Autodesk Fusion 360 part; units mm, degrees
(part 2 of 3)
  dimension "d347" = 4.5
  dimension "d348" = 4.5
  dimension "d349" = 4.5
  dimension "d350" = 4.5
  dimension "d351" = 4.5
  dimension "d352" = 4.5
  dimension "d353" = 4.5
  dimension "d354" = 4.5
  dimension "d355" = 4.5
  dimension "d356" = 4.5
  dimension "d357" = 4.5
  dimension "d358" = 4.5
  dimension "d359" = 4.5
  dimension "d360" = 4.5
  dimension "d361" = 4.5
  dimension "d362" = 4.5
  dimension "d363" = 4.5
  dimension "d364" = 4.5
  dimension "d365" = 4.5
  dimension "d366" = 4.5
  dimension "d367" = 4.5
  dimension "d368" = 4.5
  dimension "d369" = 4.5
  dimension "d370" = 4.5
  dimension "d371" = 4.5
  dimension "d372" = 4.5
  dimension "d373" = 4.5
  dimension "d374" = 4.5
  dimension "d375" = 4.5
  dimension "d376" = 4.5
  dimension "d377" = 4.5
  dimension "d378" = 4.5
  dimension "d379" = 4.5
  dimension "d380" = 4.5
  dimension "d381" = 4.5
  dimension "d382" = 4.5
  dimension "d383" = 4.5
  dimension "d384" = 4.5
  dimension "d385" = 4.5
  dimension "d386" = 4.5
  dimension "d387" = 4.5
  dimension "d388" = 4.5
  dimension "d389" = 4.5
  dimension "d390" = 4.5
  dimension "d391" = 4.5
  dimension "d392" = 4.5
  dimension "d393" = 4.5
  dimension "d394" = 4.5
  dimension "d395" = 4.5
  dimension "d396" = 4.5
  dimension "d397" = 4.5
  dimension "d398" = 4.5
  dimension "d399" = 4.5
  dimension "d400" = 4.5
  dimension "d401" = 4.5
  dimension "d402" = 4.5
  dimension "d403" = 4.5
  dimension "d404" = 4.5
  dimension "d405" = 4.5
  dimension "d406" = 4.5
  dimension "d407" = 4.5
  dimension "d408" = 4.5
  dimension "d409" = 4.5
  dimension "d410" = 4.5
  dimension "d411" = 4.5
  dimension "d412" = 4.5
  dimension "d413" = 4.5
  dimension "d414" = 4.5
  dimension "d415" = 4.5
  dimension "d416" = 4.5
  dimension "d417" = 4.5
  dimension "d418" = 4.5
  dimension "d419" = 4.5
  dimension "d420" = 4.5
  dimension "d421" = 4.5
  dimension "d422" = 4.5
  dimension "d423" = 4.5
  dimension "d424" = 4.5
  dimension "d425" = 4.5
  dimension "d426" = 4.5
  dimension "d427" = 4.5
  dimension "d428" = 4.5
  dimension "d429" = 4.5
  dimension "d430" = 4.5
  dimension "d431" = 4.5
  dimension "d432" = 4.5
  dimension "d433" = 4.5
  dimension "d434" = 4.5
  dimension "d435" = 4.5
  dimension "d436" = 4.5
  dimension "d437" = 4.5
  dimension "d438" = 4.5
  dimension "d439" = 4.5
  dimension "d440" = 4.5
  dimension "d441" = 4.5
  dimension "d442" = 4.5
  dimension "d443" = 4.5
  dimension "d444" = 4.5
  dimension "d445" = 4.5
  dimension "d446" = 4.5
  dimension "d447" = 4.5
  dimension "d448" = 4.5
  dimension "d449" = 4.5
  dimension "d450" = 4.5
  dimension "d451" = 4.5
  dimension "d452" = 4.5
  dimension "d453" = 4.5
  dimension "d454" = 4.5
  dimension "d455" = 4.5
  dimension "d456" = 4.5
  dimension "d457" = 4.5
  dimension "d458" = 4.5
  dimension "d459" = 4.5
  dimension "d460" = 4.5
  dimension "d461" = 4.5
  dimension "d462" = 4.5
  dimension "d463" = 4.5
  dimension "d464" = 4.5
  dimension "d465" = 4.5
  dimension "d466" = 4.5
  dimension "d467" = 4.5
  dimension "d468" = 4.5
  dimension "d469" = 4.5
  dimension "d470" = 4.5
  dimension "d471" = 4.5
  dimension "d472" = 4.5
  dimension "d473" = 4.5
  dimension "d474" = 4.5
  dimension "d475" = 4.5
  dimension "d476" = 4.5
  dimension "d477" = 4.5
  dimension "d478" = 4.5
  dimension "d479" = 4.5
  dimension "d480" = 4.5
  dimension "d481" = 4.5
  dimension "d482" = 4.5
  dimension "d483" = 4.5
  dimension "d484" = 4.5
  dimension "d485" = 4.5
  dimension "d486" = 4.5
  dimension "d487" = 4.5
  dimension "d488" = 4.5
  dimension "d489" = 4.5
  dimension "d490" = 4.5
  dimension "d491" = 4.5
  dimension "d492" = 4.5
  dimension "d493" = 4.5
  dimension "d494" = 4.5
  dimension "d495" = 4.5
  dimension "d496" = 4.5
  dimension "d497" = 4.5
  dimension "d498" = 4.5
  dimension "d499" = 4.5
  dimension "d500" = 4.5
  dimension "d501" = 4.5
  dimension "d502" = 4.5
  dimension "d503" = 4.5
  dimension "d504" = 4.5
  dimension "d505" = 4.5
  dimension "d506" = 4.5
  dimension "d507" = 4.5
  dimension "d508" = 4.5
  dimension "d509" = 4.5
  dimension "d510" = 4.5
  dimension "d511" = 4.5
  dimension "d512" = 4.5
  dimension "d513" = 4.5
  dimension "d514" = 75
  constraint coincident A0.centre L265.end
  constraint horizontal L0
  constraint vertical L1
  constraint horizontal L2
  constraint vertical L3
  constraint horizontal L6
  constraint vertical L4
  constraint horizontal L7
  constraint vertical L5
  constraint horizontal L12
  constraint vertical L14
  constraint horizontal L9
  constraint vertical L13
  constraint horizontal L15
  constraint vertical L8
  constraint horizontal L11
  constraint vertical L10
  constraint horizontal L20
  constraint vertical L22
  constraint horizontal L17
  constraint vertical L21
  constraint horizontal L23
  constraint vertical L16
  constraint horizontal L19
  constraint vertical L18
  constraint horizontal L28
  constraint vertical L30
  constraint horizontal L25
  constraint vertical L29
  constraint horizontal L31
  constraint vertical L24
  constraint horizontal L27
  constraint vertical L26
  constraint horizontal L36
  constraint vertical L38
  constraint horizontal L33
  constraint vertical L37
  constraint horizontal L39
  constraint vertical L32
  constraint horizontal L35
  constraint vertical L34
  constraint horizontal L44
  constraint vertical L46
  constraint horizontal L41
  constraint vertical L45
  constraint horizontal L47
  constraint vertical L40
  constraint horizontal L43
  constraint vertical L42
  constraint horizontal L52
  constraint vertical L54
  constraint horizontal L49
  constraint vertical L53
  constraint horizontal L55
  constraint vertical L48
  constraint horizontal L51
  constraint vertical L50
  constraint horizontal L86
  constraint vertical L59
  constraint horizontal L74
  constraint vertical L103
  constraint horizontal L65
  constraint vertical L78
  constraint horizontal L110
  constraint vertical L109
  constraint horizontal L94
  constraint vertical L88
  constraint horizontal L80
  constraint vertical L64
  constraint horizontal L99
  constraint vertical L58
  constraint horizontal L98
  constraint vertical L92
  constraint horizontal L87
  constraint vertical L108
  constraint horizontal L76
  constraint vertical L75
  constraint horizontal L84
  constraint vertical L77
  constraint horizontal L104
  constraint vertical L105
  constraint horizontal L111
  constraint vertical L79
  constraint horizontal L106
  constraint vertical L82
  constraint horizontal L96
  constraint vertical L81
  constraint horizontal L83
  constraint vertical L107
  constraint horizontal L97
  constraint vertical L72
  constraint horizontal L60
  constraint vertical L67
  constraint horizontal L93
  constraint vertical L66
  constraint horizontal L71
  constraint vertical L73
  constraint horizontal L101
  constraint vertical L100
  constraint horizontal L85
  constraint vertical L57
  constraint horizontal L69
  constraint vertical L102
  constraint horizontal L95
  constraint vertical L70
  constraint horizontal L56
  constraint vertical L61
  constraint horizontal L68
  constraint vertical L63
  constraint horizontal L89
  constraint vertical L90
  constraint horizontal L62
  constraint vertical L91
  constraint horizontal L223
  constraint vertical L150
  constraint horizontal L220
  constraint vertical L148
  constraint horizontal L222
  constraint vertical L141
  constraint horizontal L219
  constraint vertical L142
  constraint horizontal L217
  constraint vertical L221
  constraint horizontal L144
  constraint vertical L146
  constraint horizontal L151
  constraint vertical L211
  constraint horizontal L145
  constraint vertical L159
  constraint horizontal L186
  constraint vertical L125
  constraint horizontal L163
  constraint vertical L165
  constraint horizontal L169
  constraint vertical L210
  constraint horizontal L191
  constraint vertical L202
  constraint horizontal L137
  constraint vertical L187
  constraint horizontal L173
  constraint vertical L168
  constraint horizontal L204
  constraint vertical L164
  constraint horizontal L128
  constraint vertical L206
  constraint horizontal L215
  constraint vertical L161
  constraint horizontal L201
  constraint vertical L136
  constraint horizontal L162
  constraint vertical L147
  constraint horizontal L149
  constraint vertical L160
  constraint horizontal L209
  constraint vertical L200
  constraint horizontal L194
  constraint vertical L207
  constraint horizontal L196
  constraint vertical L214
  constraint horizontal L195
  constraint vertical L198
  constraint horizontal L130
  constraint vertical L167
  constraint horizontal L216
  constraint vertical L179
  constraint horizontal L182
  constraint vertical L193
  constraint horizontal L213
  constraint vertical L124
  constraint horizontal L114
  constraint vertical L116
  constraint horizontal L158
  constraint vertical L155
  constraint horizontal L120
  constraint vertical L118
  constraint horizontal L152
  constraint vertical L113
  constraint horizontal L112
  constraint vertical L121
  constraint horizontal L115
  constraint vertical L218
  constraint horizontal L140
  constraint vertical L177
  constraint horizontal L143
  constraint vertical L119
  constraint horizontal L170
  constraint vertical L180
  constraint horizontal L212
  constraint vertical L199
  constraint horizontal L178
  constraint vertical L185
  constraint horizontal L139
  constraint vertical L188
  constraint horizontal L129
  constraint vertical L208
  constraint horizontal L171
  constraint vertical L197
  constraint horizontal L203
  constraint vertical L205
  constraint horizontal L181
  constraint vertical L174
  constraint horizontal L122
  constraint vertical L156
  constraint horizontal L127
  constraint vertical L190
  constraint horizontal L117
  constraint vertical L153
  constraint horizontal L157
  constraint vertical L154
  constraint horizontal L131
  constraint vertical L189
  constraint horizontal L184
  constraint vertical L175
  constraint horizontal L126
  constraint vertical L123
  constraint horizontal L138
  constraint vertical L192
  constraint horizontal L135
  constraint vertical L134
  constraint horizontal L172
  constraint vertical L166
  constraint horizontal L176
  constraint vertical L133
  constraint horizontal L132
  constraint vertical L183
  constraint horizontal L439
  constraint vertical L440
  constraint horizontal L441
  constraint vertical L438
  constraint horizontal L281
  constraint vertical L300
  constraint horizontal L283
  constraint vertical L359
  constraint horizontal L289
  constraint vertical L290
  constraint horizontal L293
  constraint vertical L291
  constraint horizontal L240
  constraint vertical L430
  constraint horizontal L249
  constraint vertical L286
  constraint horizontal L434
  constraint vertical L389
  constraint horizontal L326
  constraint vertical L413
  constraint horizontal L421
  constraint vertical L385
  constraint horizontal L333
  constraint vertical L402
  constraint horizontal L376
  constraint vertical L375
  constraint horizontal L379
  constraint vertical L399
  constraint horizontal L428
  constraint vertical L373
  constraint horizontal L361
  constraint vertical L327
  constraint horizontal L356
  constraint vertical L312
  constraint horizontal L323
  constraint vertical L241
  constraint horizontal L314
  constraint vertical L311
  constraint horizontal L315
  constraint vertical L310
  constraint horizontal L239
  constraint vertical L229
  constraint horizontal L253
  constraint vertical L368
  constraint horizontal L230
  constraint vertical L244
  constraint horizontal L237
  constraint vertical L248
  constraint horizontal L391
  constraint vertical L362
  constraint horizontal L369
  constraint vertical L410
  constraint horizontal L403
  constraint vertical L423
  constraint horizontal L435
  constraint vertical L386
  constraint horizontal L437
  constraint vertical L447
  constraint horizontal L442
  constraint vertical L360
  constraint horizontal L287
  constraint vertical L301
  constraint horizontal L277
  constraint vertical L446
  constraint horizontal L282
  constraint vertical L298
  constraint horizontal L279
  constraint vertical L288
  constraint horizontal L228
  constraint vertical L396
  constraint horizontal L235
  constraint vertical L270
  constraint horizontal L426
  constraint vertical L348
  constraint horizontal L401
  constraint vertical L416
  constraint horizontal L432
  constraint vertical L397
  constraint horizontal L336
  constraint vertical L394
  constraint horizontal L387
  constraint vertical L366
  constraint horizontal L324
  constraint vertical L425
  constraint horizontal L343
  constraint vertical L380
  constraint horizontal L388
  constraint vertical L384
  constraint horizontal L352
  constraint vertical L309
  constraint horizontal L357
  constraint vertical L243
  constraint horizontal L254
  constraint vertical L255
  constraint horizontal L313
  constraint vertical L308
  constraint horizontal L227
  constraint vertical L226
  constraint horizontal L245
  constraint vertical L407
  constraint horizontal L233
  constraint vertical L234
  constraint horizontal L242
  constraint vertical L247
  constraint horizontal L427
  constraint vertical L424
  constraint horizontal L415
  constraint vertical L429
  constraint horizontal L371
  constraint vertical L414
  constraint horizontal L372
  constraint vertical L367
  constraint horizontal L445
  constraint vertical L269
  constraint horizontal L224
  constraint vertical L443
  constraint horizontal L280
  constraint vertical L305
  constraint horizontal L284
  constraint vertical L265
  constraint horizontal L296
  constraint vertical L307
  constraint horizontal L295
  constraint vertical L306
  constraint horizontal L236
  constraint vertical L345
  constraint horizontal L329
  constraint vertical L302
  constraint horizontal L404
  constraint vertical L408
  constraint horizontal L349
  constraint vertical L422
  constraint horizontal L342
  constraint vertical L420
  constraint horizontal L355
  constraint vertical L418
  constraint horizontal L365
  constraint vertical L411
  constraint horizontal L383
  constraint vertical L363
  constraint horizontal L395
  constraint vertical L364
  constraint horizontal L381
  constraint vertical L374
  constraint horizontal L334
  constraint vertical L358
  constraint horizontal L350
  constraint vertical L231
  constraint horizontal L264
  constraint vertical L256
  constraint horizontal L261
  constraint vertical L258
  constraint horizontal L419
  constraint vertical L285
  constraint horizontal L431
  constraint vertical L339
  constraint horizontal L250
  constraint vertical L278
  constraint horizontal L272
  constraint vertical L273
  constraint horizontal L340
  constraint vertical L406
  constraint horizontal L398
  constraint vertical L320
  constraint horizontal L331
  constraint vertical L351
  constraint horizontal L405
  constraint vertical L400
  constraint horizontal L268
  constraint vertical L444
  constraint horizontal L225
  constraint vertical L266
  constraint horizontal L276
  constraint vertical L297
  constraint horizontal L275
  constraint vertical L267
  constraint horizontal L292
  constraint vertical L303
  constraint horizontal L294
  constraint vertical L299
  constraint horizontal L238
  constraint vertical L321
  constraint horizontal L354
  constraint vertical L304
  constraint horizontal L392
  constraint vertical L346
  constraint horizontal L344
  constraint vertical L409
  constraint horizontal L316
  constraint vertical L412
  constraint horizontal L332
  constraint vertical L335
  constraint horizontal L390
  constraint vertical L377
  constraint horizontal L370
  constraint vertical L378
  constraint horizontal L433
  constraint vertical L382
  constraint horizontal L417
  constraint vertical L393
  constraint horizontal L318
  constraint vertical L263
  constraint horizontal L347
  constraint vertical L271
  constraint horizontal L257
  constraint vertical L259
  constraint horizontal L260
  constraint vertical L262
  constraint horizontal L325
  constraint vertical L246
  constraint horizontal L436
  constraint vertical L330
  constraint horizontal L232
  constraint vertical L251
  constraint horizontal L252
  constraint vertical L274
  constraint horizontal L322
  constraint vertical L319
  constraint horizontal L328
  constraint vertical L317
  constraint horizontal L338
  constraint vertical L337
  constraint horizontal L341
  constraint vertical L353
  constraint horizontal L663
  constraint vertical L664
  constraint horizontal L665
  constraint vertical L662
  constraint horizontal L505
  constraint vertical L524
  constraint horizontal L507
  constraint vertical L583
  constraint horizontal L513
  constraint vertical L514
  constraint horizontal L517
  constraint vertical L515
  constraint horizontal L464
  constraint vertical L654
  constraint horizontal L473
  constraint vertical L510
  constraint horizontal L658
  constraint vertical L613
  constraint horizontal L550
  constraint vertical L637
  constraint horizontal L645
  constraint vertical L609
  constraint horizontal L557
  constraint vertical L626
  constraint horizontal L600
  constraint vertical L599
  constraint horizontal L603
  constraint vertical L623
  constraint horizontal L652
  constraint vertical L597
  constraint horizontal L585
  constraint vertical L551
  constraint horizontal L580
  constraint vertical L536
  constraint horizontal L547
  constraint vertical L465
  constraint horizontal L538
  constraint vertical L535
  constraint horizontal L539
  constraint vertical L534
  constraint horizontal L463
  constraint vertical L453
  constraint horizontal L477
  constraint vertical L592
  constraint horizontal L454
  constraint vertical L468
  constraint horizontal L461
  constraint vertical L472
  constraint horizontal L615
  constraint vertical L586
  constraint horizontal L593
  constraint vertical L634
  constraint horizontal L627
  constraint vertical L647
  constraint horizontal L659
  constraint vertical L610
  constraint horizontal L661
  constraint vertical L671
  constraint horizontal L666
  constraint vertical L584
  constraint horizontal L511
  constraint vertical L525
  constraint horizontal L501
  constraint vertical L670
  constraint horizontal L506
  constraint vertical L522
  constraint horizontal L503
  constraint vertical L512
  constraint horizontal L452
  constraint vertical L620
  constraint horizontal L459
  constraint vertical L494
  constraint horizontal L650
  constraint vertical L572
  constraint horizontal L625
  constraint vertical L640
  constraint horizontal L656
  constraint vertical L621
  constraint horizontal L560
  constraint vertical L618
  constraint horizontal L611
  constraint vertical L590
  constraint horizontal L548
  constraint vertical L649
  constraint horizontal L567
  constraint vertical L604
  constraint horizontal L612
  constraint vertical L608
  constraint horizontal L576
  constraint vertical L533
  constraint horizontal L581
  constraint vertical L467
  constraint horizontal L478
  constraint vertical L479
  constraint horizontal L537
  constraint vertical L532
  constraint horizontal L451
  constraint vertical L450
  constraint horizontal L469
  constraint vertical L631
  constraint horizontal L457
  constraint vertical L458
  constraint horizontal L466
  constraint vertical L471
  constraint horizontal L651
  constraint vertical L648
  constraint horizontal L639
  constraint vertical L653
  constraint horizontal L595
  constraint vertical L638
  constraint horizontal L596
  constraint vertical L591
  constraint horizontal L669
  constraint vertical L493
  constraint horizontal L448
  constraint vertical L667
  constraint horizontal L504
  constraint vertical L529
  constraint horizontal L508
  constraint vertical L489
  constraint horizontal L520
  constraint vertical L531
  constraint horizontal L519
  constraint vertical L530
  constraint horizontal L460
  constraint vertical L569
  constraint horizontal L553
  constraint vertical L526
  constraint horizontal L628
  constraint vertical L632
  constraint horizontal L573
  constraint vertical L646
  constraint horizontal L566
  constraint vertical L644
  constraint horizontal L579
  constraint vertical L642
  constraint horizontal L589
  constraint vertical L635
  constraint horizontal L607
  constraint vertical L587
  constraint horizontal L619
  constraint vertical L588
  constraint horizontal L605
  constraint vertical L598
  constraint horizontal L558
  constraint vertical L582
  constraint horizontal L574
  constraint vertical L455
  constraint horizontal L488
  constraint vertical L480
  constraint horizontal L485
  constraint vertical L482
  constraint horizontal L643
  constraint vertical L509
  constraint horizontal L655
  constraint vertical L563
  constraint horizontal L474
  constraint vertical L502
  constraint horizontal L496
  constraint vertical L497
  constraint horizontal L564
  constraint vertical L630
  constraint horizontal L622
  constraint vertical L544
  constraint horizontal L555
  constraint vertical L575
  constraint horizontal L629
  constraint vertical L624
  constraint horizontal L492
  constraint vertical L668
  constraint horizontal L449
  constraint vertical L490
  constraint horizontal L500
  constraint vertical L521
  constraint horizontal L499
  constraint vertical L491
  constraint horizontal L516
  constraint vertical L527
  constraint horizontal L518
  constraint vertical L523
  constraint horizontal L462
  constraint vertical L545
  constraint horizontal L578
  constraint vertical L528
  constraint horizontal L616
  constraint vertical L570
  constraint horizontal L568
  constraint vertical L633
  constraint horizontal L540
  constraint vertical L636
  constraint horizontal L556
  constraint vertical L559
  constraint horizontal L614
  constraint vertical L601
  constraint horizontal L594
  constraint vertical L602
  constraint horizontal L657
  constraint vertical L606
  constraint horizontal L641
  constraint vertical L617
  constraint horizontal L542
  constraint vertical L487
  constraint horizontal L571
  constraint vertical L495
  constraint horizontal L481
  constraint vertical L483
  constraint horizontal L484
  constraint vertical L486
  constraint horizontal L549
  constraint vertical L470
  constraint horizontal L660
  constraint vertical L554
  constraint horizontal L456
  constraint vertical L475
  constraint horizontal L476
  constraint vertical L498
  constraint horizontal L546
  constraint vertical L543
  constraint horizontal L552
  constraint vertical L541
  constraint horizontal L562
  constraint vertical L561
  constraint horizontal L565
  constraint vertical L577
  constraint horizontal L887
  constraint vertical L888
  constraint horizontal L889
  constraint vertical L886
  constraint horizontal L729
  constraint vertical L748
  constraint horizontal L731
  constraint vertical L807
  constraint horizontal L737
  constraint vertical L738
  constraint horizontal L741
  constraint vertical L739
  constraint horizontal L688
  constraint vertical L878
  constraint horizontal L697
  constraint vertical L734
  constraint horizontal L882
  constraint vertical L837
  constraint horizontal L774
  constraint vertical L861
  constraint horizontal L869
  constraint vertical L833
  constraint horizontal L781
  constraint vertical L850
  constraint horizontal L824
  constraint vertical L823
  constraint horizontal L827
  constraint vertical L847
  constraint horizontal L876
  constraint vertical L821
  constraint horizontal L809
  constraint vertical L775
  constraint horizontal L804
  constraint vertical L760
  constraint horizontal L771
  constraint vertical L689
  constraint horizontal L762
  constraint vertical L759
  constraint horizontal L763
  constraint vertical L758
  constraint horizontal L687
  constraint vertical L677
  constraint horizontal L701
  constraint vertical L816
  constraint horizontal L678
  constraint vertical L692
  constraint horizontal L685
  constraint vertical L696
  constraint horizontal L839
  constraint vertical L810
  constraint horizontal L817
  constraint vertical L858
  constraint horizontal L851
  constraint vertical L871
  constraint horizontal L883
  constraint vertical L834
  constraint horizontal L885
  constraint vertical L895
  constraint horizontal L890
  constraint vertical L808
  constraint horizontal L735
  constraint vertical L749
  constraint horizontal L725
  constraint vertical L894
  constraint horizontal L730
  constraint vertical L746
  constraint horizontal L727
  constraint vertical L736
  constraint horizontal L676
  constraint vertical L844
  constraint horizontal L683
  constraint vertical L718
  constraint horizontal L874
  constraint vertical L796
  constraint horizontal L849
  constraint vertical L864
  constraint horizontal L880
  constraint vertical L845
  constraint horizontal L784
  constraint vertical L842
  constraint horizontal L835
  constraint vertical L814
  constraint horizontal L772
  constraint vertical L873
  constraint horizontal L791
  constraint vertical L828
  constraint horizontal L836
  constraint vertical L832
  constraint horizontal L800
  constraint vertical L757
  constraint horizontal L805
  constraint vertical L691
  constraint horizontal L702
  constraint vertical L703
  constraint horizontal L761
  constraint vertical L756
  constraint horizontal L675
  constraint vertical L674
  constraint horizontal L693
  constraint vertical L855
  constraint horizontal L681
  constraint vertical L682
  constraint horizontal L690
  constraint vertical L695
  constraint horizontal L875
  constraint vertical L872
  constraint horizontal L863
  constraint vertical L877
  constraint horizontal L819
  constraint vertical L862
  constraint horizontal L820
  constraint vertical L815
  constraint horizontal L893
  constraint vertical L717
  constraint horizontal L672
  constraint vertical L891
  constraint horizontal L728
  constraint vertical L753
  constraint horizontal L732
  constraint vertical L713
  constraint horizontal L744
  constraint vertical L755
  constraint horizontal L743
  constraint vertical L754
  constraint horizontal L684
  constraint vertical L793
  constraint horizontal L777
  constraint vertical L750
  constraint horizontal L852
  constraint vertical L856
  constraint horizontal L797
  constraint vertical L870
  constraint horizontal L790
  constraint vertical L868
  constraint horizontal L803
  constraint vertical L866
  constraint horizontal L813
  constraint vertical L859
  constraint horizontal L831
  constraint vertical L811
  constraint horizontal L843
  constraint vertical L812
  constraint horizontal L829
  constraint vertical L822
  constraint horizontal L782
  constraint vertical L806
  constraint horizontal L798
  constraint vertical L679
  constraint horizontal L712
  constraint vertical L704
  constraint horizontal L709
  constraint vertical L706
  constraint horizontal L867
  constraint vertical L733
  constraint horizontal L879
  constraint vertical L787
  constraint horizontal L698
  constraint vertical L726
  constraint horizontal L720
  constraint vertical L721
  constraint horizontal L788
  constraint vertical L854
  constraint horizontal L846
  constraint vertical L768
  constraint horizontal L779
  constraint vertical L799
  constraint horizontal L853
  constraint vertical L848
  constraint horizontal L716
  constraint vertical L892
  constraint horizontal L673
  constraint vertical L714
  constraint horizontal L724
  constraint vertical L745
  constraint horizontal L723
  constraint vertical L715
  constraint horizontal L740
  constraint vertical L751
  constraint horizontal L742
  constraint vertical L747
  constraint horizontal L686
  constraint vertical L769
  constraint horizontal L802
  constraint vertical L752
  constraint horizontal L840
  constraint vertical L794
  constraint horizontal L792
  constraint vertical L857
  constraint horizontal L764
  constraint vertical L860
  constraint horizontal L780
  constraint vertical L783
  constraint horizontal L838
  constraint vertical L825
  constraint horizontal L818
  constraint vertical L826
  constraint horizontal L881
  constraint vertical L830
  constraint horizontal L865
  constraint vertical L841
  constraint horizontal L766
  constraint vertical L711
  constraint horizontal L795
  constraint vertical L719
  constraint horizontal L705
  constraint vertical L707
  constraint horizontal L708
  constraint vertical L710
  constraint horizontal L773
  constraint vertical L694
  constraint horizontal L884
  constraint vertical L778
  constraint horizontal L680
  constraint vertical L699
  constraint horizontal L700
  constraint vertical L722
  constraint horizontal L770
  constraint vertical L767
  constraint horizontal L776
  constraint vertical L765
  constraint horizontal L786
  constraint vertical L785
  constraint horizontal L789
  constraint vertical L801
  constraint horizontal L935
  constraint vertical L933
  constraint horizontal L940
  constraint vertical L915
  constraint horizontal L896
  constraint vertical L921
  constraint horizontal L919
  constraint vertical L941
  constraint horizontal L928
  constraint vertical L905
  constraint horizontal L918
  constraint vertical L927
  constraint horizontal L925
  constraint vertical L908
  constraint horizontal L909
  constraint vertical L902
  constraint horizontal L907
  constraint vertical L900
  constraint horizontal L926
  constraint vertical L917
  constraint horizontal L912
  constraint vertical L903
  constraint horizontal L901
  constraint vertical L899
  constraint horizontal L913
  constraint vertical L911
  constraint horizontal L897
  constraint vertical L914
  constraint horizontal L898
  constraint vertical L904
  constraint horizontal L906
  constraint vertical L910
  constraint horizontal L932
  constraint vertical L943
  constraint horizontal L934
  constraint vertical L937
  constraint horizontal L936
  constraint vertical L939
  constraint horizontal L931
  constraint vertical L938
  constraint horizontal L946
  constraint vertical L949
  constraint horizontal L929
  constraint vertical L950
  constraint horizontal L922
  constraint vertical L942
  constraint horizontal L924
  constraint vertical L948
  constraint horizontal L945
  constraint vertical L920
  constraint horizontal L951
  constraint vertical L930
  constraint horizontal L944
  constraint vertical L947
  constraint horizontal L923
  constraint vertical L916
  constraint horizontal L991
  constraint vertical L989
  constraint horizontal L996
  constraint vertical L971
  constraint horizontal L952
  constraint vertical L977
  constraint horizontal L975
  constraint vertical L997
  constraint horizontal L984
  constraint vertical L961
  constraint horizontal L974
  constraint vertical L983
  constraint horizontal L981
  constraint vertical L964
  constraint horizontal L965
  constraint vertical L958
  constraint horizontal L963
  constraint vertical L956
  constraint horizontal L982
  constraint vertical L973
  constraint horizontal L968
  constraint vertical L959
  constraint horizontal L957
  constraint vertical L955
  constraint horizontal L969
  constraint vertical L967
  constraint horizontal L953
  constraint vertical L970
  constraint horizontal L954
  constraint vertical L960
  constraint horizontal L962
  constraint vertical L966
  constraint horizontal L988
  constraint vertical L999
  constraint horizontal L990
  constraint vertical L993
  constraint horizontal L992
  constraint vertical L995
  constraint horizontal L987
  constraint vertical L994
  constraint horizontal L1002
  constraint vertical L1005
  constraint horizontal L985
  constraint vertical L1006
  constraint horizontal L978
  constraint vertical L998
  constraint horizontal L980
  constraint vertical L1004
  constraint horizontal L1001
  constraint vertical L976
  constraint horizontal L1007
  constraint vertical L986
  constraint horizontal L1000
  constraint vertical L1003
  constraint horizontal L979
  constraint vertical L972
  constraint horizontal L1008
  constraint vertical L1009
  constraint horizontal L1010
  constraint vertical L1011
  measures "d10" distance of L0.start L0.end
  measures "d11" distance of L0.start L2.end
  measures "d12" distance of L4.start L5.end
  measures "d13" distance of L5.start L5.end
  measures "d14" distance of L12.end L12.start
  measures "d15" distance of L9.end L12.start
  measures "d16" distance of L10.end L8.start
  measures "d17" distance of L10.start L10.end
  measures "d18" distance of L20.end L20.start
  measures "d19" distance of L17.end L20.start
  measures "d20" distance of L18.end L16.start
  measures "d21" distance of L18.start L18.end
  measures "d22" distance of L28.end L28.start
  measures "d23" distance of L25.end L28.start
  measures "d24" distance of L26.end L24.start
  measures "d25" distance of L26.start L26.end
  measures "d26" distance of L36.end L36.start
  measures "d27" distance of L33.end L36.start
  measures "d28" distance of L34.end L32.start
  measures "d29" distance of L34.start L34.end
  measures "d30" distance of L44.end L44.start
  measures "d31" distance of L41.end L44.start
  measures "d32" distance of L42.end L40.start
  measures "d33" distance of L42.start L42.end
  measures "d34" distance of L52.end L52.start
  measures "d35" distance of L49.end L52.start
  measures "d36" distance of L50.end L48.start
  measures "d37" distance of L50.start L50.end
  measures "d38" distance of L59.start L86.start
  measures "d39" distance of L74.end L86.start
  measures "d40" distance of L65.start L65.end
  measures "d41" distance of L109.start L65.start
  measures "d42" distance of L64.end L88.start
  measures "d43" distance of L64.end L64.start
  measures "d44" distance of L58.start L92.end
  measures "d45" distance of L92.start L92.end
  measures "d46" distance of L87.end L75.end
  measures "d47" distance of L75.start L75.end
  measures "d48" distance of L84.start L77.start
  measures "d49" distance of L104.end L84.start
  measures "d50" distance of L82.end L79.start
  measures "d51" distance of L82.start L82.end
  measures "d52" distance of L96.start L81.start
  measures "d53" distance of L83.end L96.start
  measures "d54" distance of L67.end L72.start
  measures "d55" distance of L67.end L60.end
  measures "d56" distance of L73.end L66.start
  measures "d57" distance of L73.end L71.end
  measures "d58" distance of L100.start L57.end
  measures "d59" distance of L57.start L57.end
  measures "d60" distance of L69.end L69.start
  measures "d61" distance of L69.start L70.start
  measures "d62" distance of L56.end L56.start
  measures "d63" distance of L63.start L56.start
  measures "d64" distance of L89.start L89.end
  measures "d65" distance of L89.start L62.end
  measures "d66" distance of L150.start L148.end
  measures "d67" distance of L148.start L148.end
  measures "d68" distance of L142.end L141.start
  measures "d69" distance of L142.start L142.end
  measures "d70" distance of L146.end L217.end
  measures "d71" distance of L146.end L144.end
  measures "d72" distance of L151.end L151.start
  measures "d73" distance of L145.end L151.start
  measures "d74" distance of L125.start L165.end
  measures "d75" distance of L163.end L165.end
  measures "d76" distance of L169.start L169.end
  measures "d77" distance of L191.end L169.start
  measures "d78" distance of L137.start L137.end
  measures "d79" distance of L168.start L137.start
  measures "d80" distance of L204.start L164.start
  measures "d81" distance of L128.end L204.start
  measures "d82" distance of L136.end L161.start
  measures "d83" distance of L136.end L136.start
  measures "d84" distance of L160.end L147.start
  measures "d85" distance of L160.end L149.end
  measures "d86" distance of L200.start L207.end
  measures "d87" distance of L194.end L207.end
  measures "d88" distance of L196.end L196.start
  measures "d89" distance of L196.start L195.end
  measures "d90" distance of L130.end L130.start
  measures "d91" distance of L179.start L130.start
  measures "d92" distance of L124.end L182.end
  measures "d93" distance of L124.end L124.start
  measures "d94" distance of L114.end L114.start
  measures "d95" distance of L155.start L114.start
  measures "d96" distance of L118.start L113.end
  measures "d97" distance of L113.start L113.end
  measures "d98" distance of L112.end L112.start
  measures "d99" distance of L112.start L115.end
  measures "d100" distance of L140.end L119.end
  measures "d101" distance of L119.start L119.end
  measures "d102" distance of L170.end L170.start
  measures "d103" distance of L199.start L170.start
  measures "d104" distance of L178.start L178.end
  measures "d105" distance of L139.end L178.start
  measures "d106" distance of L129.end L129.start
  measures "d107" distance of L171.end L129.start
  measures "d108" distance of L203.end L174.end
  measures "d109" distance of L174.start L174.end
  measures "d110" distance of L122.start L122.end
  measures "d111" distance of L122.start L127.end
  measures "d112" distance of L117.start L117.end
  measures "d113" distance of L117.start L154.start
  measures "d114" distance of L131.end L131.start
  measures "d115" distance of L175.start L131.start
  measures "d116" distance of L126.start L123.start
  measures "d117" distance of L126.start L138.end
  measures "d118" distance of L135.start L134.start
  measures "d119" distance of L135.start L166.start
  measures "d120" distance of L176.start L133.start
  measures "d121" distance of L176.start L132.end
  measures "d122" distance of L439.end L438.end
  measures "d123" distance of L438.start L438.end
  measures "d124" distance of L281.start L281.end
  measures "d125" distance of L283.end L281.start
  measures "d126" distance of L289.start L289.end
  measures "d127" distance of L289.start L291.start
  measures "d128" distance of L240.end L240.start
  measures "d129" distance of L249.end L240.start
  measures "d130" distance of L389.start L413.end
  measures "d131" distance of L326.end L413.end
  measures "d132" distance of L402.end L385.start
  measures "d133" distance of L333.end L402.end
  measures "d134" distance of L376.start L375.start
  measures "d135" distance of L379.end L376.start
  measures "d136" distance of L327.end L373.start
  measures "d137" distance of L327.start L327.end
  measures "d138" distance of L241.end L312.start
  measures "d139" distance of L241.end L241.start
  measures "d140" distance of L310.end L311.start
  measures "d141" distance of L310.end L310.start
  measures "d142" distance of L229.start L239.start
  measures "d143" distance of L253.end L239.start
  measures "d144" distance of L230.end L230.start
  measures "d145" distance of L230.start L237.end
  measures "d146" distance of L362.start L391.start
  measures "d147" distance of L369.end L391.start
  measures "d148" distance of L386.end L403.end
  measures "d149" distance of L386.end L386.start
  measures "d150" distance of L437.end L360.end
  measures "d151" distance of L360.start L360.end
  measures "d152" distance of L287.end L287.start
  measures "d153" distance of L277.end L287.start
  measures "d154" distance of L282.end L282.start
  measures "d155" distance of L282.start L279.end
  measures "d156" distance of L228.end L228.start
  measures "d157" distance of L235.end L228.start
  measures "d158" distance of L348.start L416.end
  measures "d159" distance of L401.end L416.end
  measures "d160" distance of L394.end L397.start
  measures "d161" distance of L336.end L394.end
  measures "d162" distance of L366.start L387.start
  measures "d163" distance of L324.end L387.start
  measures "d164" distance of L343.end L343.start
  measures "d165" distance of L384.start L343.start
  measures "d166" distance of L243.end L309.start
  measures "d167" distance of L243.end L243.start
  measures "d168" distance of L254.start L254.end
  measures "d169" distance of L254.start L308.start
  measures "d170" distance of L226.start L227.start
  measures "d171" distance of L245.end L227.start
  measures "d172" distance of L233.start L233.end
  measures "d173" distance of L233.start L242.end
  measures "d174" distance of L427.start L424.start
  measures "d175" distance of L427.start L415.end
  measures "d176" distance of L367.end L371.end
  measures "d177" distance of L367.end L367.start
  measures "d178" distance of L443.end L269.start
  measures "d179" distance of L224.end L443.end
  measures "d180" distance of A0.centre L280.end
  measures "d181" distance of A0.centre L265.start
  measures "d182" distance of L296.end L296.start
  measures "d183" distance of L295.end L296.start
  measures "d184" distance of L236.end L236.start
  measures "d185" distance of L302.start L236.start
  measures "d186" distance of L404.start L404.end
  measures "d187" distance of L404.start L349.end
  measures "d188" distance of L342.start L342.end
  measures "d189" distance of L342.start L355.end
  measures "d190" distance of L365.end L363.end
  measures "d191" distance of L363.end L363.start
  measures "d192" distance of L364.start L374.end
  measures "d193" distance of L374.end L374.start
  measures "d194" distance of L231.end L334.end
  measures "d195" distance of L231.start L231.end
  measures "d196" distance of L258.end L256.start
  measures "d197" distance of L258.end L258.start
  measures "d198" distance of L285.start L339.end
  measures "d199" distance of L339.end L339.start
  measures "d200" distance of L250.end L250.start
  measures "d201" distance of L272.end L250.start
  measures "d202" distance of L320.end L340.end
  measures "d203" distance of L320.end L320.start
  measures "d204" distance of L331.start L331.end
  measures "d205" distance of L331.start L400.start
  measures "d206" distance of L268.end L266.end
  measures "d207" distance of L225.end L266.end
  measures "d208" distance of L276.end L267.end
  measures "d209" distance of L267.start L267.end
  measures "d210" distance of L292.start L292.end
  measures "d211" distance of L292.start L294.end
  measures "d212" distance of L238.end L238.start
  measures "d213" distance of L238.start L304.start
  measures "d214" distance of L346.start L392.start
  measures "d215" distance of L344.end L392.start
  measures "d216" distance of L316.start L316.end
  measures "d217" distance of L332.end L316.start
  measures "d218" distance of L378.end L377.start
  measures "d219" distance of L378.end L370.end
  measures "d220" distance of L393.end L382.start
  measures "d221" distance of L393.end L393.start
  measures "d222" distance of L271.end L263.start
  measures "d223" distance of L271.end L271.start
  measures "d224" distance of L257.end L257.start
  measures "d225" distance of L260.end L257.start
  measures "d226" distance of L246.start L325.start
  measures "d227" distance of L330.start L325.start
  measures "d228" distance of L232.end L232.start
  measures "d229" distance of L232.start L252.end
  measures "d230" distance of L319.start L317.end
  measures "d231" distance of L317.start L317.end
  measures "d232" distance of L337.start L338.start
  measures "d233" distance of L341.end L338.start
  measures "d234" distance of L0.end L0.start
  measures "d235" distance of L2.end L0.start
  measures "d236" distance of L5.end L4.start
  measures "d237" distance of L5.start L5.end
  measures "d238" distance of L12.start L12.end
  measures "d239" distance of L12.start L9.end
  measures "d240" distance of L8.start L10.end
  measures "d241" distance of L10.start L10.end
  measures "d242" distance of L20.end L20.start
  measures "d243" distance of L17.end L20.start
  measures "d244" distance of L18.end L16.start
  measures "d245" distance of L18.start L18.end
  measures "d246" distance of L28.start L28.end
  measures "d247" distance of L25.end L28.start
  measures "d248" distance of L26.end L24.start
  measures "d249" distance of L26.start L26.end
  measures "d250" distance of L36.start L36.end
  measures "d251" distance of L36.start L33.end
  measures "d252" distance of L34.end L32.start
  measures "d253" distance of L34.end L34.start
  measures "d254" distance of L44.end L44.start
  measures "d255" distance of L41.end L44.start
  measures "d256" distance of L40.start L42.end
  measures "d257" distance of L42.end L42.start
  measures "d258" distance of L52.end L52.start
  measures "d259" distance of L49.end L52.start
  measures "d260" distance of L50.end L48.start
  measures "d261" distance of L50.end L50.start
  measures "d262" distance of L59.start L86.start
  measures "d263" distance of L74.end L86.start
  measures "d264" distance of L65.end L65.start
  measures "d265" distance of L109.start L65.start
  measures "d266" distance of L88.start L64.end
  measures "d267" distance of L64.end L64.start
  measures "d268" distance of L58.start L92.end
  measures "d269" distance of L92.start L92.end
  measures "d270" distance of L87.end L75.end
  measures "d271" distance of L75.start L75.end
  measures "d272" distance of L84.start L77.start
  measures "d273" distance of L104.end L84.start
  measures "d274" distance of L79.start L82.end
  measures "d275" distance of L82.start L82.end
  measures "d276" distance of L81.start L96.start
  measures "d277" distance of L83.end L96.start
  measures "d278" distance of L67.end L72.start
  measures "d279" distance of L67.end L60.end
  measures "d280" distance of L73.end L66.start
  measures "d281" distance of L73.end L71.end
  measures "d282" distance of L100.start L57.end
  measures "d283" distance of L57.start L57.end
  measures "d284" distance of L69.start L69.end
  measures "d285" distance of L69.start L70.start
  measures "d286" distance of L56.start L56.end
  measures "d287" distance of L56.start L63.start
  measures "d288" distance of L89.start L89.end
  measures "d289" distance of L89.start L62.end
  measures "d290" distance of L148.end L150.start
  measures "d291" distance of L148.start L148.end
  measures "d292" distance of L142.end L141.start
  measures "d293" distance of L142.end L142.start
  measures "d294" distance of L217.end L146.end
  measures "d295" distance of L144.end L146.end
  measures "d296" distance of L151.end L151.start
  measures "d297" distance of L145.end L151.start
  measures "d298" distance of L165.end L125.start
  measures "d299" distance of L165.end L163.end
  measures "d300" distance of L169.start L169.end
  measures "d301" distance of L169.start L191.end
  measures "d302" distance of L137.end L137.start
  measures "d303" distance of L137.start L168.start
  measures "d304" distance of L164.start L204.start
  measures "d305" distance of L204.start L128.end
  measures "d306" distance of L136.end L161.start
  measures "d307" distance of L136.start L136.end
  measures "d308" distance of L160.end L147.start
  measures "d309" distance of L160.end L149.end
  measures "d310" distance of L200.start L207.end
  measures "d311" distance of L207.end L194.end
  measures "d312" distance of L196.end L196.start
  measures "d313" distance of L195.end L196.start
  measures "d314" distance of L130.start L130.end
  measures "d315" distance of L130.start L179.start
  measures "d316" distance of L124.end L182.end
  measures "d317" distance of L124.end L124.start
  measures "d318" distance of L114.end L114.start
  measures "d319" distance of L155.start L114.start
  measures "d320" distance of L118.start L113.end
  measures "d321" distance of L113.start L113.end
  measures "d322" distance of L112.start L112.end
  measures "d323" distance of L112.start L115.end
  measures "d324" distance of L140.end L119.end
  measures "d325" distance of L119.end L119.start
  measures "d326" distance of L170.end L170.start
  measures "d327" distance of L199.start L170.start
  measures "d328" distance of L178.start L178.end
  measures "d329" distance of L139.end L178.start
  measures "d330" distance of L129.start L129.end
  measures "d331" distance of L129.start L171.end
  measures "d332" distance of L174.end L203.end
  measures "d333" distance of L174.end L174.start
  measures "d334" distance of L122.start L122.end
  measures "d335" distance of L122.start L127.end
  measures "d336" distance of L117.end L117.start
  measures "d337" distance of L154.start L117.start
  measures "d338" distance of L131.end L131.start
  measures "d339" distance of L175.start L131.start
  measures "d340" distance of L123.start L126.start
  measures "d341" distance of L126.start L138.end
  measures "d342" distance of L134.start L135.start
  measures "d343" distance of L166.start L135.start
  measures "d344" distance of L133.start L176.start
  measures "d345" distance of L132.end L176.start
  measures "d346" distance of L887.end L886.end
  measures "d347" distance of L886.start L886.end
  measures "d348" distance of L729.start L729.end
  measures "d349" distance of L731.end L729.start
  measures "d350" distance of L737.start L737.end
  measures "d351" distance of L737.start L739.start
  measures "d352" distance of L688.end L688.start
  measures "d353" distance of L697.end L688.start
  measures "d354" distance of L837.start L861.end
  measures "d355" distance of L774.end L861.end
  measures "d356" distance of L850.end L833.start
  measures "d357" distance of L781.end L850.end
  measures "d358" distance of L824.start L823.start
  measures "d359" distance of L827.end L824.start
  measures "d360" distance of L775.end L821.start
  measures "d361" distance of L775.start L775.end
  measures "d362" distance of L689.end L760.start
  measures "d363" distance of L689.end L689.start